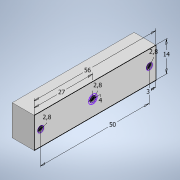
# Autodesk Inventor part: AdaptadorSensorWSMotionPart2
Saved by Autodesk Inventor 2020.3 (Build 243373000, 373)
## iProperties
Created: 2020-09-09
Part Number: AdaptadorSensorWSMotionPart2
Material: Generic
Document SubType Name: Modeling
Designer: mifer
Density: 1 g/cm^3
Appearance: Default
Author: mifer
## iProperties of the stored document _3DPrint.ipt
Created: 2020-09-09
Part Number: _3DPrint
Material: Generic
Document SubType Name: Modeling
Designer: mifer
Density: 1 g/cm^3
Appearance: Default
Author: mifer
Autodesk Inventor part; units mm, degrees
ref_plane "YZ Plane" through (0, 0, 0) normal (1, 0, 0) x (0, 1, 0)
ref_plane "XZ Plane" through (0, 0, 0) normal (0, 1, 0) x (-1, 0, 0)
ref_plane "XY Plane" through (0, 0, 0) normal (0, 0, 1) x (1, 0, 0)
sketch "Sketch1" plane through (0, 0, 0) normal (1, 0, 0) x (0, 1, 0)
  line L0 (0, 0) -> (14, 0)
  line L1 (14, 0) -> (14, -56)
  line L2 (14, -56) -> (0, -56)
  line L3 (0, -56) -> (0, 0)
  circle A0 centre (7, -27) radius 1.4
  circle A1 centre (7, -27) radius 2
  circle A2 centre (7, -3) radius 1.4
  circle A3 centre (7, -53) radius 1.4
  dimension "d0" = 56
  dimension "d1" = 14
  dimension "d2" = 2.8
  dimension "d3" = 4
  dimension "d4" = 27
  dimension "d5" = 2.8
  dimension "d6" = 2.8
  dimension "d7" = 50
  dimension "d8" = 3
  constraints: 8 end point, 4 centre point, 2 parallel, 1 coincident, 1 horizontal, 1 perpendicular
  measures "d0" distance of L0.end L1.end
  measures "d1" distance of L1.end L2.end
  measures "d2" diameter of A0
  measures "d3" diameter of A1
  measures "d4" distance from line of L0 A0.centre
  measures "d5" diameter of A2
  measures "d6" diameter of A3
  measures "d7" distance of A3.centre A2.centre
  measures "d8" distance from line of L2 A3.centre
extrude "Extrusion1" add sketch "Sketch1" against normal blind 10 contours L0 L1 L2 L3
extrude "Extrusion2" add sketch "Sketch1" against normal blind 6 contours A1
body "Solid1"
